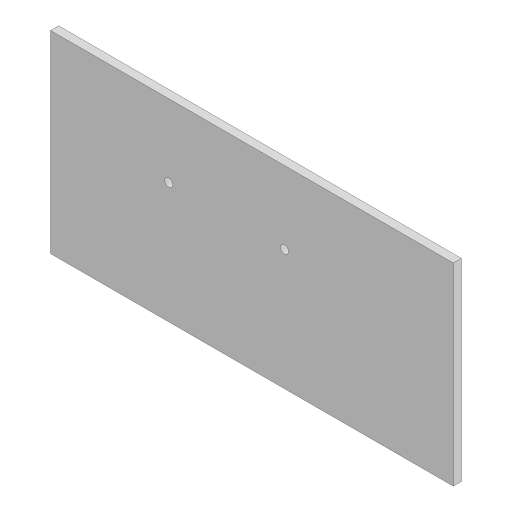
# Autodesk Inventor part: team29_wall
Saved by Autodesk Inventor 2023 (Build 270158000, 158)
## iProperties
Created: 2023-03-05
Part Number: team29_wall
Material: Generic
Document SubType Name: Modeling
Designer: Ethan Ko
Density: 1 g/cm^3
Appearance: Default
Author: Ethan Ko
Autodesk Inventor part; units mm, degrees
ref_plane "YZ Plane" through (0, 0, 0) normal (1, 0, 0) x (0, 1, 0)
ref_plane "XZ Plane" through (0, 0, 0) normal (0, 1, 0) x (-1, 0, 0)
ref_plane "XY Plane" through (0, 0, 0) normal (0, 0, 1) x (1, 0, 0)
sketch "Sketch1" plane through (0, 0, 0) normal (0, 0, 1) x (1, 0, 0)
  line L0 (0, 0) -> (250, 0)
  line L1 (250, 0) -> (250, 120)
  line L2 (250, 120) -> (0, 120)
  line L3 (0, 120) -> (0, 0)
  dimension "d0" = 250
  dimension "d1" = 120
  constraints: 8 end point, 2 parallel, 1 horizontal, 1 perpendicular
  measures "d0" distance of L2.end L1.end
  measures "d1" distance of L1.end L0.end
extrude "Extrusion1" add sketch "Sketch1" along normal blind 5
sketch "Sketch2" plane through (0, 0, 5) normal (0, 0, 1) x (1, 0, 0)
  circle A0 centre (73.3331, 74.9591) radius 2.5
  circle A1 centre (145.2027, 74.9591) radius 2.5
  point P0 (0, 0)
  dimension "d4" = 5
  dimension "d5" = 5
  constraints: 2 centre point
  measures "d4" diameter of A0
  measures "d5" diameter of A1
extrude "Extrusion2" cut sketch "Sketch2" against normal blind 5
body "Solid1"
